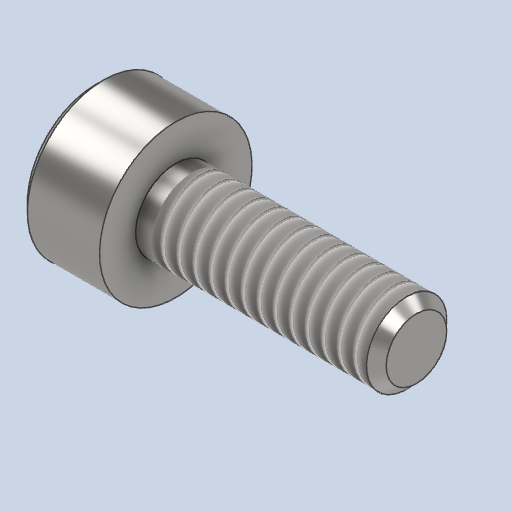
# Autodesk Inventor part: BOLT2-6
Saved by Autodesk Inventor 2023 (Build 270158000, 158)
## iProperties
Category: PARTsolutions
Company: MISUMI
Created: 2024-12-13
Part Number: BOLT2-6
Material: ステンレス鋼
Catalog Web Link: www.cadenas.de
Description: BOLT-Hexagon Socket Head Cap Screws
Vendor: MISUMI
Document SubType Name: Modeling
Designer: psAdmin
Manufacturer: MISUMI
Mass: 0.312486 g
Surface Area: 0.870833 cm^2
Volume: 0.0390607 cm^3
Density: 8 g/cm^3
Appearance: 半つや出し
PSOL_IDENT_0: {$CADENAS_DATA/23d-libs/misumi/metric/accessories/bolt.prj},155 {VTYP=3D},{NB=BOLT2-6},{LINA=BOLT2-6
PSOL_IDENT_1: },{NN=BOLT},{DATE=29.11.2024 04:47:06},{GEOMDATE=12.05.2017 08:21:09},{VERSION=},{LINEID=210},{WBVAR=
PSOL_IDENT_2: L},{WBNUMERIC=L}  {NB=BOLT2-6},{LINA=BOLT2-6},{KT=DUMMY},{PN=BOLT2-6},{TYPE=BOLT},{L=6.0},{M=2.0},{P=
PSOL_IDENT_3: 0.4},{A=3.8},{E=2.0},{B=1.5},{C=0.20},{LL=0}
NB: BOLT2-6
NN: BOLT
NT: Hexagon Socket Head Cap Screws
NBSYN: $PN.
LINA: BOLT2-6
CATALOG: Misumi
PN: BOLT2-6
L: 6
M: 2
P: 0.4
C: 0.2
SUPPLIER: MISUMI
ARTICLENO: BOLT2-6
BOMINFO: BOLT2-6
CREATOR: CADENAS GmbH
Title: BOLT2-6
Author: Cadenas PARTsolutions
Comments: Hexagon Socket Head Cap Screws
Autodesk Inventor part; units mm, degrees
sketch "Sketch_1" plane through (0, 0, 0) normal (0, 0, 1) x (1, 0, 0)
  line L0 (6, 0) -> (-2, 0)
  line L1 (-2, 0) -> (-2, 1.7)
  line L2 (-2, 1.7) -> (-1.8, 1.9)
  line L3 (-1.8, 1.9) -> (0, 1.9)
  line L4 (0, 1.9) -> (0, 1)
  line L5 (0, 1) -> (5.7545, 1)
  line L6 (5.7545, 1) -> (6, 0.7545)
  line L7 (6, 0.7545) -> (6, 0)
  line L8 (6, 0) -> (-2, 0)
  constraints: 18 end point
revolve "Revolution1" add sketch "Sketch_1" angle 360 about axis through (6, 0, 0) along (1, 0, 0)
thread "Thread1" size "M2x0.4" class "6g" standard "ISO Metric profile" length 5.3545
sketch "Sketch2" plane through (-2, 0, 0) normal (-1, 0, 0) x (0, 0, 1)
  point P0 (0, 0)
hole "Hole1" at (-2, 0, 0) direction (1, 0, 0) diameter 1.5 depth 1 tip angle 150
sketch "Sketch_3" plane through (-2, 0, 0) normal (1, 0, 0) x (0, 0, -1)
  line L0 (-0.75, -0.433) -> (0, -0.866)
  line L1 (0, -0.866) -> (0.75, -0.433)
  line L2 (0.75, -0.433) -> (0.75, 0.433)
  line L3 (0.75, 0.433) -> (0, 0.866)
  line L4 (0, 0.866) -> (-0.75, 0.433)
  line L5 (-0.75, 0.433) -> (-0.75, -0.433)
  constraints: 12 end point
extrude "Extrusion1" cut sketch "Sketch_3" along normal blind 1
ref_plane "to_cp_XY" through (0, 0, 0) normal (1, 0, 0) x (0, 0, -1)
ref_plane "to_cp_YZ" through (0, 0, 0) normal (0, 0, -1) x (0, 1, 0)
ref_plane "to_cp_ZX" through (0, 0, 0) normal (0, 1, 0) x (1, 0, 0)
body "Solid1"
